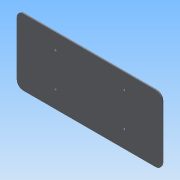
# Autodesk Inventor part: Plate
Saved by Autodesk Inventor 2014 (Build 180170000, 170)
## iProperties
Created: 2012-05-24
Part Number: Plate
Material: Generic
Document SubType Name: Modeling
Designer: dgitz
Density: 1 g/cm^3
Appearance: Steel
Author: dgitz
Autodesk Inventor part; units mm, degrees
ref_plane "YZ Plane" through (0, 0, 0) normal (1, 0, 0) x (0, 1, 0)
ref_plane "XZ Plane" through (0, 0, 0) normal (0, 1, 0) x (-1, 0, 0)
ref_plane "XY Plane" through (0, 0, 0) normal (0, 0, 1) x (1, 0, 0)
sketch "Sketch1" plane through (0, 0, 0) normal (0, 0, 1) x (1, 0, 0)
  line L0 (-107.95, 49.53) -> (107.95, 49.53)
  line L1 (107.95, 49.53) -> (107.95, -49.53)
  line L2 (107.95, -49.53) -> (-107.95, -49.53)
  line L3 (-107.95, -49.53) -> (-107.95, 49.53)
  line L4 (-107.95, 49.53) -> (107.95, -49.53) construction
  point P0 (0, 0)
  point P1 (0, 0)
  dimension "d0" = 99.06
  dimension "d1" = 215.9
  constraints: 10 end point, 2 parallel, 1 coincident, 1 horizontal, 1 midpoint, 1 perpendicular
  measures "d0" distance between parallel lines of L2 L0
  measures "d1" distance of L0.start L0.end
extrude "Extrusion1" add sketch "Sketch1" along normal mid plane 1.778
fillet "Fillet1" radius 9.525 4 edges at (107.95, 49.53, 0) (107.95, -49.53, 0) (-107.95, 49.53, 0) (-107.95, -49.53, 0)
sketch "Sketch2" plane through (0, 0, -0.889) normal (0, 0, -1) x (-1, 0, 0)
  line L0 (107.95, 40.005) -> (107.95, -40.005) projected
  line L1 (-98.425, 49.53) -> (98.425, 49.53) projected
  line L2 (-107.95, -40.005) -> (-107.95, 40.005) projected
  line L3 (98.425, -49.53) -> (-98.425, -49.53) projected
  circle A0 centre (-51.4096, 26.416) radius 1.5875
  circle A1 centre (50.8, 26.416) radius 1.5875
  circle A2 centre (-51.4096, -23.876) radius 1.5875
  circle A3 centre (50.8, -23.876) radius 1.5875
  line L4 (-51.4096, 26.416) -> (50.8, 26.416) construction
  line L5 (50.8, 26.416) -> (50.8, -23.876) construction
  line L6 (50.8, -23.876) -> (-51.4096, -23.876) construction
  line L7 (-51.4096, -23.876) -> (-51.4096, 26.416) construction
  point P0 (0, 0)
  dimension "d5" = 56.5404
  dimension "d6" = 23.114
  dimension "d7" = 25.654
  dimension "d8" = 57.15
  dimension "d9" = 3.175
  constraints: 8 end point, 4 centre point, 3 equal radius, 3 perpendicular, 1 parallel
  measures "d5" distance from line of L4.start L2
  measures "d6" distance between parallel lines of L1 L4
  measures "d7" distance between parallel lines of L3 L6
  measures "d8" distance between parallel lines of L0 L5
  measures "d9" diameter of A0
extrude "Extrusion2" cut sketch "Sketch2" against normal up to next
body "Solid1"
